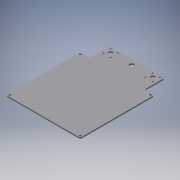
# Autodesk Inventor part: Byggeplade Holder mk2
Saved by Autodesk Inventor 2016 (Build 200138000, 138)
## iProperties
Created: 2015-10-17
Part Number: Byggeplade Holder mk2
Material: Generic
Document SubType Name: Modeling
Designer: iLyngklip
Density: 1 g/cm^3
Appearance: Default
Author: iLyngklip
Autodesk Inventor part; units mm, degrees
ref_plane "YZ Plane" through (0, 0, 0) normal (1, 0, 0) x (0, 1, 0)
ref_plane "XZ Plane" through (0, 0, 0) normal (0, 1, 0) x (-1, 0, 0)
ref_plane "XY Plane" through (0, 0, 0) normal (0, 0, 1) x (1, 0, 0)
sketch "Sketch1" plane through (0, 0, 0) normal (0, 0, 1) x (1, 0, 0)
  line L0 (-115, 145.15) -> (115, 145.15)
  line L1 (115, 145.15) -> (115, -145.15)
  line L2 (115, -145.15) -> (-115, -145.15)
  line L3 (-115, -145.15) -> (-115, 145.15)
  line L4 (-115, 145.15) -> (-85, 145.15)
  line L5 (-85, 145.15) -> (-85, 84.85)
  line L6 (-85, 84.85) -> (-115, 84.85)
  line L7 (-115, 84.85) -> (-115, 145.15)
  line L8 (115, 145.15) -> (85, 145.15)
  line L9 (85, 145.15) -> (85, 84.85)
  line L10 (85, 84.85) -> (115, 84.85)
  line L11 (115, 84.85) -> (115, 145.15)
  circle A0 centre (-65, 129.15) radius 6.5
  circle A1 centre (65, 129.15) radius 6.5
  circle A2 centre (0, 129.15) radius 6
  line L12 (65, 129.15) -> (-65, 129.15) construction
  circle A3 centre (-109, 78.85) radius 3
  circle A4 centre (109, 78.85) radius 3
  circle A5 centre (109, -139.15) radius 3
  circle A6 centre (-109, -139.15) radius 3
  line L13 (109, -139.15) -> (-109, -139.15) construction
  line L14 (109, -139.15) -> (109, 78.85) construction
  line L15 (-109, 78.85) -> (-109, -139.15) construction
  line L16 (109, 78.85) -> (-109, 78.85) construction
  point P0 (0, 0)
  dimension "d0" = 290.3
  dimension "d1" = 230
  dimension "d2" = 30
  dimension "d3" = 30
  dimension "d4" = 60.3
  dimension "d5" = 13
  dimension "d6" = 13
  dimension "d7" = 12
  dimension "d8" = 130
  dimension "d9" = 65
  dimension "d10" = 16
  dimension "d11" = 6
  dimension "d12" = 6
  dimension "d13" = 6
  dimension "d14" = 6
  dimension "d15" = 218
  dimension "d16" = 218
  dimension "d17" = 218
  dimension "d18" = 218
  dimension "d19" = 115
  dimension "d20" = 145.15
  dimension "d21" = 6
  dimension "d22" = 6
  constraints: 34 end point, 7 centre point, 6 parallel, 5 horizontal, 3 perpendicular, 1 midpoint, 1 point on line, 1 vertical
  measures "d0" distance of L0.end L1.end
  measures "d1" distance of L1.end L2.end
  measures "d2" distance of L5.end L6.end
  measures "d3" distance of L9.end L10.end
  measures "d4" distance of L4.end L5.end
  measures "d5" diameter of A1
  measures "d6" diameter of A0
  measures "d7" diameter of A2
  measures "d8" distance of L12.start L12.end
  measures "d9" horizontal distance of L12.end point (0, 0)
  measures "d10" distance from line of L0 L12.end
  measures "d11" diameter of A6
  measures "d12" diameter of A5
  measures "d13" diameter of A4
  measures "d14" diameter of A3
  measures "d15" distance of L14.end L13.start
  measures "d16" distance of L15.start L13.end
  measures "d17" distance of L13.end L13.start
  measures "d18" distance of L15.start L14.end
  measures "d19" distance from line of point (0, 0) L1
  measures "d20" distance from line of point (0, 0) L2
  measures "d21" distance between parallel lines of L2 L13
  measures "d22" distance between parallel lines of L1 L14
extrude "Tykkelse" add sketch "Sketch1" along normal mid plane 4 contours L0 L9 L10 L1 L2 L3 L6 L5
fillet "Fillet1" radius 6 4 edges at (115, -145.15, 0) (-115, -145.15, 0) (-115, 84.85, 0) (115, 84.85, 0)
fillet "Fillet2" radius 3 4 edges at (-85, 84.85, 0) (-85, 145.15, 0) (85, 84.85, 0) (85, 145.15, 0)
sketch "Sketch2" plane through (0, 0, 2) normal (0, 0, 1) x (1, 0, 0)
  line L0 (78, 145.15) -> (81, 142.15) projected
  line L1 (78, 145.15) -> (52, 145.15) projected
  line L2 (49, 142.15) -> (52, 145.15) projected
  line L3 (49, 142.15) -> (49, 116.15) projected
  line L4 (52, 113.15) -> (49, 116.15) projected
  line L5 (52, 113.15) -> (78, 113.15) projected
  line L6 (81, 116.15) -> (78, 113.15) projected
  line L7 (81, 116.15) -> (81, 142.15) projected
  circle A0 centre (53.6863, 140.4637) radius 2.25 projected
  circle A1 centre (53.6863, 117.8363) radius 2.25 projected
  circle A2 centre (76.3137, 140.4637) radius 2.25 projected
  circle A3 centre (76.3137, 117.8363) radius 2.25 projected
  circle A4 centre (65, 129.15) radius 10.5 projected
  line L8 (-81, 142.15) -> (-78, 145.15) projected
  line L9 (-81, 142.15) -> (-81, 116.15) projected
  line L10 (-78, 113.15) -> (-81, 116.15) projected
  line L11 (-78, 113.15) -> (-52, 113.15) projected
  line L12 (-49, 116.15) -> (-52, 113.15) projected
  line L13 (-49, 116.15) -> (-49, 142.15) projected
  line L14 (-52, 145.15) -> (-49, 142.15) projected
  line L15 (-52, 145.15) -> (-78, 145.15) projected
  circle A5 centre (-76.3137, 117.8363) radius 2.25 projected
  circle A6 centre (-53.6863, 117.8363) radius 2.25 projected
  circle A7 centre (-76.3137, 140.4637) radius 2.25 projected
  circle A8 centre (-53.6863, 140.4637) radius 2.25 projected
  circle A9 centre (-65, 129.15) radius 10.5 projected
  point P0 (0, 0)
extrude "Flange-huller" cut sketch "Sketch2" against normal blind 10 contours A0 | A1 | A2 | A3 | A5 | A6 | A7 | A8
sketch "Sketch3" plane through (0, 0, 2) normal (0, 0, 1) x (1, 0, 0)
  circle A0 centre (0, 129.15) radius 4 construction
  circle A1 centre (0, 121.15) radius 0.75
  circle A2 centre (0, 137.15) radius 0.75
  circle A3 centre (-8, 129.15) radius 0.75
  circle A4 centre (8, 129.15) radius 0.75
  line L0 (0, 137.15) -> (0, 121.15) construction
  line L1 (-8, 129.15) -> (8, 129.15) construction
  circle A5 centre (7.954, 128.2933) radius 0.9464 construction
  circle A6 centre (0, 129.15) radius 8 construction
  point P0 (0, 0)
  dimension "d29" = 1.5
  constraints: 5 centre point, 4 end point, 3 equal radius, 2 coincident, 2 midpoint, 2 perpendicular, 2 point on circle, 1 vertical
  measures "d29" diameter of A4
extrude "Flange møtrik" cut sketch "Sketch3" against normal blind 10
equation "\"d3\" = d2"
equation "\"d6\" = d5"
equation "\"d9\" = 0.5 * d8"
equation "\"d12\" = d11"
equation "\"d13\" = d11"
equation "\"d14\" = d11"
equation "\"d19\" = 0.5 * d1"
equation "\"d20\" = 0.5 * d0"
body "Solid1"
